Autodesk Fusion 360 part; units mm, degrees
(part 2 of 2)
extrude "돌출3'" add sketch "스케치2 (6)" along normal blind 9 contours A2 bodies 6 in component "TRGRIP01_Case_Top"
sketch "스케치4 (3)" plane through (0, 0, 11) normal (0, 0, 1) x (-1, 0, 0) in component "TRGRIP01_Case_Top"
  circle A0 centre (-15, -8.1) radius 2.3
  circle A1 centre (-15, -8.1) radius 5
  dimension "d34" = 4.6
  constraint concentric A0 A1
  measures "d34" diameter of A0
extrude "돌출5'" add sketch "스케치4 (3)" along normal blind 2 contours A0 bodies 6 in component "TRGRIP01_Case_Top"
sketch "스케치5 (3)" plane through (0, 0, 2) normal (0, 0, 1) x (-1, 0, 0) in component "TRGRIP01_Case_Top"
  line L0 (0, -30) -> (0, 0)
  line L1 (0, 0) -> (0, -30)
  line L2 (-60, -30) -> (0, -30)
  line L3 (-60, -30) -> (-60, 0)
  line L4 (0, 0) -> (-60, 0)
  line L5 (-60, 0) -> (-54, 0)
  line L6 (-54, -28) -> (-6, -28)
  line L7 (-2, -24) -> (-2, -6)
  line L8 (-6, 0) -> (0, 0)
  line L9 (-58, -24) -> (-58, -6)
  line L10 (-2, -24) -> (-6, -24)
  line L11 (-6, -24) -> (-6, -28)
  line L12 (-54, -28) -> (-54, -24)
  line L13 (-54, -24) -> (-58, -24)
  line L14 (-2, -6) -> (-6, -6)
  line L15 (0, 0) -> (-60, 0)
  line L16 (-6, -6) -> (-6, 0)
  line L17 (-58, -6) -> (-54, -6)
  line L18 (-54, -6) -> (-54, 0)
  point P0 (0, -30)
  point P1 (-60, -30)
  point P2 (-60, 0)
  dimension "d38_2" = 2
  dimension "d39_2" = 2
  dimension "d42_1" = 2
  dimension "d43_1" = 6
  dimension "d44_2" = 6
  dimension "d45_2" = 6
  dimension "d46_3" = 6
  dimension "d47_3" = 6
  constraint coincident L0.end L1.start
  constraint coincident P0 L0.start
  constraint coincident P1 L2.start
  constraint coincident P2 L3.end
  constraint coincident L4 L5.end
  constraint perpendicular L0 L5
  constraint perpendicular L0 L6
  constraint perpendicular L6 L7
  constraint perpendicular L1 L8
  constraint perpendicular L5 L9
  constraint perpendicular L7 L10
  constraint perpendicular L10 L11
  constraint perpendicular L6 L12
  constraint perpendicular L9 L13
  constraint perpendicular L7 L14
  constraint coincident L15 L8.start
  constraint perpendicular L15 L16
  constraint perpendicular L9 L17
  constraint perpendicular L4 L18
  constraint equal L10 L14
  constraint equal L11 L12
  constraint equal L13 L17
  measures "d38_2" distance of L2 L6
  measures "d39_2" distance of L3 L9
  measures "d42_1" distance of L1 L7
  measures "d43_1" distance of L0.end L8.start
  measures "d44_2" vertical distance of L0.end L14.end
  measures "d45_2" distance of P2 L5.end
  measures "d46_3" distance of L17.end L5.end
  measures "d47_3" vertical distance of P0 L10.end
extrude "돌출6" add sketch "스케치5 (3)" along normal blind 12 contours L0 L1 L2 L3 L4 L5 L6 L7 L8 L9 L10 L11 L12 L13 L14 L15 L16 L17 L18 bodies 6 in component "TRGRIP01_Case_Top"
sketch "스케치6 (2)" plane through (0, 0, 14) normal (0, 0, 1) x (-1, 0, 0) in component "TRGRIP01_Case_Top"
  circle A0 centre (-3, -27) radius 0.95
  circle A1 centre (-3, -3) radius 0.95
  circle A2 centre (-57, -27) radius 0.95
  circle A3 centre (-57, -3) radius 0.95
  dimension "d48_2" = 1.9
  dimension "d49_1" = 3
  dimension "d51_1" = 3
  dimension "d52_1" = 24
  dimension "d53_2" = 54
  constraint equal A2 A3
  constraint equal A0 A2
  constraint equal A0 A1
  constraint vertical A0.centre A1.centre
  constraint horizontal A0.centre A2.centre
  constraint vertical A2.centre A3.centre
  constraint horizontal A1.centre A3.centre
  measures "d48_2" diameter of A0
  measures "d49_1" horizontal distance of origin A1.centre
  measures "d51_1" vertical distance of origin A1.centre
  measures "d52_1" distance of A0.centre A1.centre
  measures "d53_2" distance of A0.centre A2.centre
extrude "돌출7''" cut sketch "스케치6 (2)" against normal blind 5 bodies 6 in component "TRGRIP01_Case_Top"
fillet "필렛1''" radius 3 8 edges at (60, 0, 7) (0, 0, 7) (60, 30, 7) (0, 30, 7) (54, 24, 8) (6, 24, 8) (54, 6, 8) (6, 6, 8) on bodies 6 in component "TRGRIP01_Case_Top"
fillet "필렛1''" radius 3 2 edges at (54, 0, 8) (6, 0, 8) on bodies 6 in component "TRGRIP01_Case_Top"
sketch "스케치9" plane through (0, 30, 0) normal (0, 1, 0) x (-1, 0, 0) in component "TRGRIP01_Case_Top"
  circle A0 centre (-50, 8) radius 1.5
  circle A1 centre (-30, 8) radius 1.5
  circle A2 centre (-10, 8) radius 1.5
  circle A3 centre (-40, 8) radius 1.5
  circle A4 centre (-20, 8) radius 1.5
  dimension "d74" = 3
  dimension "d75_1" = 8
  dimension "d80" = 10
  dimension "d81" = 10
  dimension "d82_1" = 10
  dimension "d83_1" = 10
  dimension "d84_1" = 10
  constraint horizontal A0.centre A1.centre
  constraint equal A0 A1
  constraint equal A1 A2
  constraint horizontal A1.centre A2.centre
  constraint equal A1 A3
  constraint equal A1 A4
  constraint horizontal A1.centre A3.centre
  constraint horizontal A3.centre A4.centre
  measures "d74" diameter of A0
  measures "d75_1" vertical distance of origin A1.centre
  measures "d80" horizontal distance of origin A2.centre
  measures "d81" distance of A2.centre A4.centre
  measures "d82_1" distance of A1.centre A4.centre
  measures "d83_1" distance of A1.centre A3.centre
  measures "d84_1" distance of A0.centre A3.centre
extrude "돌출10'" cut sketch "스케치9" against normal blind 2 bodies 6 in component "TRGRIP01_Case_Top"
sketch "스케치1 (10)" plane through (0, 0, 0) normal (0, 0, 1) x (1, 0, 0) in component "SG90"
  line L0 (0, 0) -> (23, 0)
  line L1 (23, 0) -> (23, 12)
  line L2 (23, 12) -> (0, 12)
  line L3 (0, 12) -> (0, 0)
  dimension "d1_3" = 23
  dimension "d2_3" = 12
  constraint horizontal L0
  constraint vertical L1
  constraint horizontal L2
  constraint vertical L3
  constraint coincident L0.start L3.end
  measures "d1_3" distance of L0.start L0.end
  measures "d2_3" distance of L0.start L2.end
extrude "돌출1''''''" add sketch "스케치1 (10)" along normal blind 24 separate body makes body 7 in component "SG90"
sketch "스케치2 (7)" plane through (0, 0, 0) normal (-1, 0, 0) x (0, -1, 0) in component "SG90"
  line L0 (-12, 20.5) -> (0, 20.5)
  line L1 (0, 20.5) -> (0, 18)
  line L2 (0, 18) -> (-12, 18)
  line L3 (-12, 18) -> (-12, 20.5)
  line L4 (-12, 0) -> (-12, 24)
  line L5 (0, 0) -> (0, 24)
  dimension "d9_4" = 18
  dimension "d10_3" = 2.5
  constraint horizontal L0
  constraint vertical L1
  constraint horizontal L2
  constraint vertical L3
  constraint coincident L1.end L5
  constraint coincident L0.start L4
  measures "d9_4" distance of L5.start L1.end
  measures "d10_3" distance of L0.end L1.end
extrude "돌출2''''" add sketch "스케치2 (7)" along normal blind 4.5 bodies 7 in component "SG90"
sketch "스케치3 (6)" plane through (23, 0, 0) normal (1, 0, 0) x (0, 1, 0) in component "SG90"
  line L0 (0, 20.5) -> (12, 20.5)
  line L1 (12, 20.5) -> (12, 18)
  line L2 (12, 18) -> (0, 18)
  line L3 (0, 18) -> (0, 20.5)
  line L4 (0, 18) -> (0, 20.5)
  line L5 (12, 0) -> (12, 18)
  constraint horizontal L0
  constraint vertical L1
  constraint horizontal L2
  constraint vertical L3
  constraint coincident L1.end L5
  constraint coincident L0.start L3.end
  constraint coincident L2.end L3.start
extrude "돌출3''" add sketch "스케치3 (6)" along normal blind 4.5 bodies 7 in component "SG90"
sketch "스케치4 (4)" plane through (0, 0, 20.5) normal (0, 0, 1) x (-1, 0, 0) in component "SG90"
  circle A0 centre (2.4, -6) radius 1.25
  circle A1 centre (-25.4, -6) radius 1.25
  dimension "d12_3" = 6
  dimension "d13_3" = 27.8
  dimension "d14_3" = 2.5
  dimension "d15_3" = 2.4
  constraint equal A0 A1
  constraint horizontal A0.centre A1.centre
  measures "d12_3" vertical distance of origin A0.centre
  measures "d13_3" distance of A0.centre A1.centre
  measures "d14_3" diameter of A0
  measures "d15_3" horizontal distance of origin A0.centre
extrude "돌출4" cut sketch "스케치4 (4)" against normal blind 2.5 bodies 7 in component "SG90"
sketch "스케치5 (4)" plane through (0, 0, 24) normal (0, 0, 1) x (-1, 0, 0) in component "SG90"
  arc A0 (-11.7644, -8.72) -> (-11.7644, -3.28) centre (-11.1, -6) ccw
  arc A1 (-11.7644, -3.28) -> (-11.7644, -8.72) centre (-17, -6) ccw
  dimension "d18_1" = 6
  dimension "d19_1" = 11.8
  dimension "d20_1" = 17
  dimension "d24" = 2.8
  constraint horizontal A1.centre A0.centre
  constraint coincident A0.centre A1
  measures "d18_1" vertical distance of origin A1.centre
  measures "d19_1" diameter of A1
  measures "d20_1" horizontal distance of origin A1.centre
  measures "d24" radius of A0
extrude "돌출6'" add sketch "스케치5 (4)" along normal blind 4 bodies 7 in component "SG90"
sketch "스케치6 (3)" plane through (0, 0, 28) normal (0, 0, 1) x (-1, 0, 0) in component "SG90"
  circle A0 centre (-17, -6) radius 2.5
  arc A1 (-11.7644, -3.28) -> (-11.7644, -8.72) centre (-17, -6) ccw
  dimension "d27_1" = 5
  constraint concentric A0 A1
  measures "d27_1" diameter of A0
extrude "돌출7'''" add sketch "스케치6 (3)" along normal blind 3 bodies 7 in component "SG90"
component "TRARM02_Link4A_30x40x2 v1" placed x (1, 0, 0) y (0, 1, 0) z (0, 0, 1) at (0, 0, 0)
component "TRARM02_Link4B_30x40x28 v1" placed x (0, 1, 0) y (1, 0, 0) z (0, 0, -1) at (0, 0, 30)
component "TRGRIP01_Assemble_v0.2 v1" placed x (0, 1, 0) y (-1, 0, 0) z (0, 0, 1) at (60, -30, -10)
component "TRGRIP01_Case_Bottom" placed x (1, 0, 0) y (0, 1, 0) z (0, 0, 1) at (0, 0, 0) in component "TRGRIP01_Assemble_v0.2 v1"
component "TRGRIP01_GearLink_Left" placed x (0, 1, 0) y (-1, 0, 0) z (0, 0, 1) at (87, -40, 53) in component "TRGRIP01_Assemble_v0.2 v1"
component "TRGRIP01_GearLink_Right" placed x (-0.258819, 0.965926, 0) y (-0.965926, -0.258819, 0) z (0, 0, 1) at (12.6075, -43.6063, 43) in component "TRGRIP01_Assemble_v0.2 v1"
component "TRGRIP01_Case_Top" placed x (-1, 0, 0) y (0, 1, 0) z (0, 0, -1) at (60, 0, 18) in component "TRGRIP01_Assemble_v0.2 v1"
component "SG90" placed x (-1, 0, 0) y (0, 1, 0) z (0, 0, -1) at (31.65, 2.1, 38.5) in component "TRGRIP01_Assemble_v0.2 v1"
component "Spur Gear (12 teeth)" placed x (1, 0, 0) y (0, 1, 0) z (0, 0, 1) at (0, 0, 0) in component "TRGRIP01_GearLink_Left"
component "Spur Gear (12 teeth) (1)" placed x (1, 0, 0) y (0, 1, 0) z (0, 0, 1) at (48.1, 42, -51) in component "TRGRIP01_GearLink_Left"
component "Spur Gear (12 teeth) (2)" placed x (1, 0, 0) y (0, 1, 0) z (0, 0, 1) at (0, 0, 0) in component "TRGRIP01_GearLink_Right"
component "Spur Gear (12 teeth) (1) (1)" placed x (-1, 0, 0) y (0, -1, 0) z (0, 0, 1) at (49.3252, -15.6935, -41) in component "TRGRIP01_GearLink_Right"
